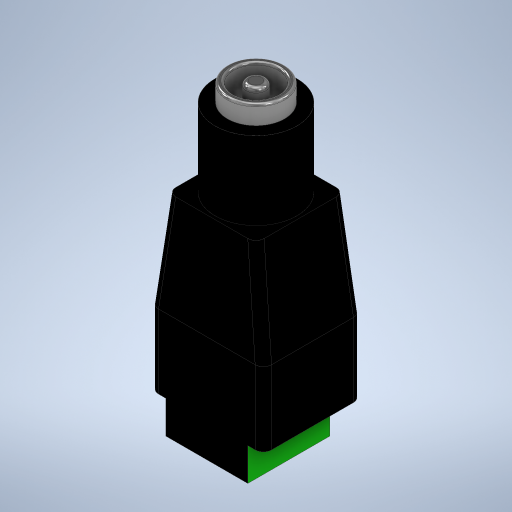
# Autodesk Inventor part: ConectorFuente
Saved by Autodesk Inventor 2024 (Build 280153000, 153)
## iProperties
Created: 2024-05-29
Part Number: ConectorFuente
Material: Genérico
Document SubType Name: Modeling
Designer: alexa
Density: 1 g/cm^3
Appearance: Valor por defecto
Author: alexa
Autodesk Inventor part; units mm, degrees
ref_plane "YZ Plane" through (0, 0, 0) normal (1, 0, 0) x (0, 1, 0)
ref_plane "XZ Plane" through (0, 0, 0) normal (0, 1, 0) x (-1, 0, 0)
sketch "Sketch1" plane through (0, 0, 0) normal (0, 1, 0) x (-1, 0, 0)
  circle A0 centre (0, 0) radius 5
  dimension "d0" = 10
  constraints: 1 centre point, 1 coincident
  measures "d0" diameter of A0
extrude "Extrusion1" add sketch "Sketch1" along normal blind 9.5
sketch "Sketch2" plane through (0, 9.5, 0) normal (0, 1, 0) x (1, 0, 0)
  circle A0 centre (0, 0) radius 3.5
  dimension "d3" = 7
  constraints: 1 centre point, 1 coincident
  measures "d3" diameter of A0
extrude "Extrusion2" add sketch "Sketch2" along normal blind 2.3
sketch "Sketch3" plane through (0, 0, 0) normal (0, -1, 0) x (1, 0, 0)
  line L0 (5.4, -5.4) -> (-5.4, -5.4)
  line L1 (-5.4, -5.4) -> (-5.4, 5.4)
  line L2 (-5.4, 5.4) -> (5.4, 5.4)
  line L3 (5.4, 5.4) -> (5.4, -5.4)
  line L4 (5.4, -5.4) -> (-5.4, 5.4) construction
  line L5 (-5.4, -5.4) -> (5.4, 5.4) construction
  point P0 (0, 0)
  dimension "d6" = 10.8
  dimension "d7" = 10.8
  constraints: 12 end point, 2 midpoint, 2 parallel, 1 horizontal, 1 perpendicular
  measures "d6" distance of L1.end L2.end
  measures "d7" distance of L0.end L1.end
ref_plane "Work Plane1" through (0, -12.3, 0) normal (0, -1, 0) x (1, 0, 0)
sketch "Sketch4" plane through (0, -12.3, 0) normal (0, -1, 0) x (1, 0, 0)
  line L0 (6.9, -6) -> (-6.9, -6)
  line L1 (-6.9, -6) -> (-6.9, 6)
  line L2 (-6.9, 6) -> (6.9, 6)
  line L3 (6.9, 6) -> (6.9, -6)
  line L4 (6.9, -6) -> (-6.9, 6) construction
  line L5 (-6.9, -6) -> (6.9, 6) construction
  point P0 (0, 0)
  dimension "d9" = 13.8
  dimension "d10" = 12
  constraints: 12 end point, 2 midpoint, 2 parallel, 1 horizontal, 1 perpendicular
  measures "d9" distance of L1.end L2.end
  measures "d10" distance of L0.end L1.end
loft "Loft1" add profiles "Sketch3", "Sketch4"
sketch "Sketch6" plane through (-6.9, -12.3, -6) normal (0, -1, 0) x (1, 0, 0)
  line L0 (12.3, 0.6) -> (13.8, 0) projected
  line L1 (0, 12) -> (13.8, 12)
  line L2 (13.8, 12) -> (13.8, 0)
  line L3 (13.8, 0) -> (0, 0)
  line L4 (0, 0) -> (0, 12)
  line L5 (0, 12) -> (13.8, 0) construction
  line L6 (13.8, 12) -> (0, 0) construction
  point P0 (6.9, 6)
  constraints: 12 end point, 2 midpoint, 2 parallel, 1 horizontal, 1 perpendicular
extrude "Extrusion3" add sketch "Sketch6" along normal blind 9
fillet "Fillet2" radius 1 8 edges at (6.15, -6.15, -5.7) (-6.15, -6.15, -5.7) (6.15, -6.15, 5.7) (-6.15, -6.15, 5.7) (6.9, -16.8, 6) (6.9, -16.8, -6) (-6.9, -16.8, 6) (-6.9, -16.8, -6)
sketch "Sketch8" plane through (-6.9, -21.3, -6) normal (0, -1, 0) x (1, 0, 0)
  line L0 (1.0015, 12) -> (12.7985, 12) projected
  line L1 (11.9, 12) -> (11.9, 2)
  line L2 (11.9, 2) -> (1.9, 2)
  line L3 (1.9, 2) -> (1.9, 12)
  line L4 (1.9, 12) -> (11.9, 12)
  line L5 (13.8, 1) -> (13.8, 11) projected
  line L6 (0, 11) -> (0, 1) projected
  point P0 (6.9, 6)
  dimension "d25" = 10
  dimension "d26" = 10
  dimension "d27" = 1.9
  dimension "d29" = 1.9
  constraints: 8 end point, 2 perpendicular, 2 point on line, 1 collinear
  measures "d25" distance of L1.start L1.end
  measures "d26" distance of L1.end L2.end
  measures "d27" distance between parallel lines of L5 L1
  measures "d29" distance between parallel lines of L6 L3
extrude "Extrusion5" add sketch "Sketch8" along normal blind 4
sketch "Sketch9" plane through (0, 11.8, 0) normal (0, 1, 0) x (1, 0, 0)
  circle A0 centre (0, 0) radius 1.175
  circle A1 centre (0, 0) radius 2.75
  dimension "d32" = 2.35
  dimension "d33" = 5.5
  constraints: 2 centre point, 2 coincident
  measures "d32" diameter of A0
  measures "d33" diameter of A1
extrude "Extrusion6" cut sketch "Sketch9" against normal blind 7.9
fillet "Fillet3" radius 0.5 1 edges at (-1.175, 11.8, 0)
fillet "Fillet4" radius 0.3 1 edges at (-3.5, 11.8, 0)
fillet "Fillet5" radius 0.3 1 edges at (-2.75, 11.8, 0)
body "Solid1"
